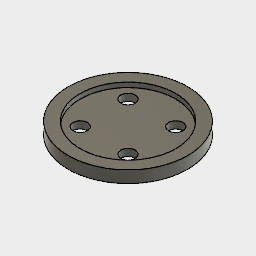
kou (Autodesk Fusion 360 design; units mm, degrees)
Autodesk Fusion 360 part; units mm, degrees
sketch "草图1" plane through (0, 0, 0) normal (0, 1, 0) x (1, 0, 0)
  circle A0 centre (0, 0) radius 25
extrude "拉伸1" add sketch "草图1" along normal blind 5
sketch "草图2" plane through (0, 5, 0) normal (0, 1, 0) x (-1, 0, 0)
  circle A0 centre (0, 0) radius 25
  circle A1 centre (0, 0) radius 20
extrude "拉伸2" cut sketch "草图2" against normal blind 2 contours A1
sketch "草图3" plane through (0, 3, 0) normal (0, 1, 0) x (-1, 0, 0)
  circle A0 centre (0, 0) radius 20
  circle A1 centre (7.861, -8.3613) radius 4.4141
cylinder "圆柱体基本要素1" cut diameter 6 height -10 placed x (1, 0, 0) y (0, 0, -1) z (0, 1, 0) at (-10, 3, -10)
cylinder "圆柱体基本要素2" cut diameter 6 height -8 placed x (1, 0, 0) y (0, 0, -1) z (0, 1, 0) at (10, 3, -10)
cylinder "圆柱体基本要素3" cut diameter 6 height -6 placed x (1, 0, 0) y (0, 0, -1) z (0, 1, 0) at (-10, 3, 10)
cylinder "圆柱体基本要素4" cut diameter 6 height -5 placed x (1, 0, 0) y (0, 0, -1) z (0, 1, 0) at (10, 3, 10)
extrude "拉伸3" [suppressed]
